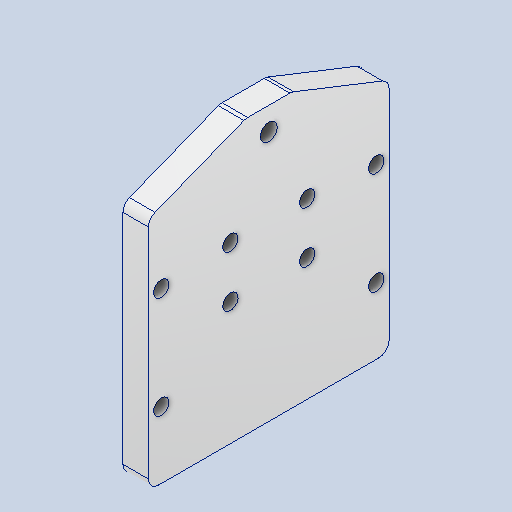
# Autodesk Inventor part: odom_v1_Plate_2
Saved by Autodesk Inventor 2025.2 (Build 292293000, 293)
## iProperties
Created: 2025-03-30
Part Number: odom_v1_Plate_2
Material: アルミニウム 6061
Document SubType Name: Modeling
Designer: haruy
Density: 2.7 g/cm^3
Appearance: アルミニウム - フラット
Author: haruy
Autodesk Inventor part; units mm, degrees
ref_plane "YZ Plane" through (0, 0, 0) normal (1, 0, 0) x (0, 1, 0)
ref_plane "XZ Plane" through (0, 0, 0) normal (0, 1, 0) x (-1, 0, 0)
ref_plane "XY Plane" through (0, 0, 0) normal (0, 0, 1) x (1, 0, 0)
derived "odom_v1_Sketch_Base.ipt"
sketch "スケッチ1" plane through (300, 0, 0) normal (1, 0, 0) x (0, 1, 0)
  line L0 (0, 0) -> (20, 0)
  line L1 (20, 0) -> (20, -192.6893)
  line L2 (20, -192.6893) -> (0, -192.6893)
  line L3 (0, -192.6893) -> (0, 0)
  line L4 (-77, 0) -> (-77, -265.1297)
  circle A0 centre (7.5, -57.9764) radius 1.6
  circle A1 centre (7.5, -93.4764) radius 1.6
  line L5 (-20, -52.2264) -> (-66, -52.2264)
  line L6 (-66, -52.2264) -> (-66, -57.2264)
  line L7 (-66, -57.2264) -> (-20, -57.2264)
  line L8 (-20, -57.2264) -> (-20, -52.2264)
  line L9 (-20, -94.2264) -> (-66, -94.2264)
  line L10 (-66, -94.2264) -> (-66, -99.2264)
  line L11 (-66, -99.2264) -> (-20, -99.2264)
  line L12 (-20, -99.2264) -> (-20, -94.2264)
  line L13 (-19.371, -66.7264) -> (-77, -66.7264)
  line L14 (-77, -66.7264) -> (-77, -84.7264)
  line L15 (-77, -84.7264) -> (-19.371, -84.7264)
  line L16 (-19.371, -84.7264) -> (-19.371, -66.7264)
  line L17 (-41.1855, -57.2264) -> (-55.1855, -57.2264)
  line L18 (-55.1855, -57.2264) -> (-55.1855, -58.0264)
  line L19 (-55.1855, -58.0264) -> (-41.1855, -58.0264)
  line L20 (-41.1855, -58.0264) -> (-41.1855, -57.2264)
  line L21 (-48.1855, -66.7264) -> (-48.1855, -84.7264)
  line L22 (-55.1855, -94.2264) -> (-41.1855, -94.2264)
  line L23 (-41.1855, -94.2264) -> (-41.1855, -93.4264)
  line L24 (-41.1855, -93.4264) -> (-55.1855, -93.4264)
  line L25 (-55.1855, -93.4264) -> (-55.1855, -94.2264)
  circle A2 centre (48, -75.7264) radius 1.65
  circle A3 centre (-17, -75.7264) radius 2 construction
  line L26 (48, -75.7264) -> (-17, -75.7264)
  line L27 (33.5, -67.2264) -> (-12, -67.2264)
  line L28 (-12, -67.2264) -> (-12, -84.2264)
  line L29 (-12, -84.2264) -> (33.5, -84.2264)
  line L30 (33.5, -84.2264) -> (33.5, -67.2264)
  line L31 (-12, -73.7264) -> (-20, -73.7264)
  line L32 (-20, -73.7264) -> (-20, -77.7264)
  line L33 (-20, -77.7264) -> (-12, -77.7264)
  line L34 (-12, -77.7264) -> (-12, -73.7264)
  line L35 (-2, -71.2264) -> (-57, -71.2264)
  line L36 (-57, -71.2264) -> (-57, -80.2264)
  line L37 (-57, -80.2264) -> (-2, -80.2264)
  line L38 (-2, -80.2264) -> (-2, -71.2264)
  circle A4 centre (-9.5, -75.7264) radius 1.25
  circle A5 centre (-29.5, -75.7264) radius 1.25
  circle A6 centre (-49.5, -75.7264) radius 1.25
  line L39 (-52, -65.7264) -> (-22, -65.7264)
  line L40 (-22, -65.7264) -> (-22, -85.7264)
  line L41 (-22, -85.7264) -> (-52, -85.7264)
  line L42 (-52, -85.7264) -> (-52, -65.7264)
  line L43 (-43, -52.2264) -> (-43, -57.2264)
  circle A7 centre (-33, -54.7264) radius 1.5
  line L44 (-29.5, -75.7264) -> (-49.5, -75.7264)
  circle A8 centre (-53, -54.7264) radius 1.5
  circle A9 centre (-53, -96.7264) radius 1.5
  circle A10 centre (-33, -96.7264) radius 1.5
  circle A11 centre (-32, -68.2264) radius 1.5
  line L45 (-37, -65.7264) -> (-37, -85.7264)
  circle A12 centre (-42, -68.2264) radius 1.5
  circle A13 centre (-32, -83.2264) radius 1.5
  circle A14 centre (-42, -83.2264) radius 1.5
  line L46 (-20, -57.2264) -> (-20, -94.2264)
  line L47 (-66, -57.2264) -> (-66, -94.2264)
  circle A15 centre (-17, -75.7264) radius 1.65
  circle A16 centre (-17, -75.7264) radius 7
  line L48 (-17, -68.7264) -> (-20, -68.7264)
  line L49 (-17, -82.7264) -> (-20, -82.7264)
  line L50 (-12.5, -71.2264) -> (-12.5, -80.2264)
  line L51 (-20, -52.2264) -> (-12.5, -71.2264)
  line L52 (-12.5, -80.2264) -> (-20, -99.2264)
  point P0 (-20, -71.2264)
  point P1 (-20, -80.2264)
  dimension "d1" = 3
  dimension "d2" = 10
  dimension "d3" = 2.5
  dimension "d6" = 3.3
  dimension "d7" = 5
  dimension "d8" = 0.5
  measures "d1" diameter of A11
  measures "d2" distance from line of A11.centre L40
  measures "d3" distance from line of A11.centre L39
  measures "d6" diameter of A15
  measures "d7" radial gap between concentric circles of A3 A16
  measures "d8" distance between parallel lines of L50 L28
extrude "押し出し1" add sketch "スケッチ1" against normal blind 5 contours L51 L35 L16 A16 | A16 L48 L16 L13 L46 L8 L51 | L50 L31 L16 L35 | A16 L16 L48 | L8 L7 L43 L5 | L52 L12 L46 L15 L16 L49 A16 | A16 L16 L37 L52 | L50 L33 L16 L31 | L35 L46 A16 L16 | L16 L31 L46 L35 | A16 L46 L48 L16 | L48 L46 L13 L16 | L43 L7 L6 L5 | L46 L13 L40 L39 L42 L47 L7 L18 L19 L20 | L37 L16 L33 L50 | L49 L16 A16 | L11 L10 L9 L12 | L16 L33 L32 L31 | L46 L32 L37 L40 L35 | L35 L40 A16 L46 | A16 L40 L13 L46 | L7 L20 L19 L18 | L37 L46 L33 L16 | L16 A16 L46 L37 | L16 L49 L46 A16 | L16 L15 L46 L49 | L9 L23 L24 L25 L47 L15 L42 L41 L40 L46 | L40 L37 A16 L35 | L35 A16 L40 | A16 L35 L45 L13 L40 | L13 L45 L39 L40 | L46 A16 L40 L37 | L46 L15 L40 A16 | L9 L25 L24 L23 | A16 L37 L45 L35 | L40 A16 L37 | L13 L42 L35 L36 L37 L15 L47 | L40 L15 L45 L37 A16 | L40 L41 L45 L15 | L45 L44 L21 L35 | L35 L21 L13 L45 | L42 L39 L45 L13 | L13 L21 L35 L42 | L42 L37 L21 L15 | L15 L45 L41 L42 | L21 L37 L42 L35 | L45 L37 L21 L44 | L45 L15 L21 L37 | L42 L37 L36 L35 | A5 | A6
fillet "フィレット1" radius 2 6 edges at (297.5, -66, -52.2264) (297.5, -66, -99.2264) (297.5, -20, -99.2264) (297.5, -12.5, -80.2264) (297.5, -12.5, -71.2264) (297.5, -20, -52.2264)
